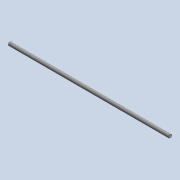
# Autodesk Inventor part: SFR6-284
Saved by Autodesk Inventor 2022 (Build 260153000, 153)
## iProperties
Part Number: SFR6-284
Material: 一般
Catalog Web Link: www.cadenas.de
Description: NSFMR, SFMR, PSFMR, SSFMR, SSSFMR, NSFHR, SFHR, PSFHR, PPSFHR SSFHR, SSSFHR, NSFR, SFR, PSFR, PPSFR, SSFR, SSSFR, HFR, PHFR_shaft-Rotary Shafts - Straight -
Vendor: MISUMI
Document SubType Name: Modeling
Designer: partserver
Manufacturer: MISUMI
Mass: 8.02546 g
Surface Area: 53.9813 cm^2
Volume: 8.02546 cm^3
Density: 1 g/cm^3
Appearance: PSOLRGB-192-192-192
Category: PARTsolutions
Company: MISUMI
PSOL_IDENT_0: {$CADENAS_DATA\23d-libs\misumi\metric\11_rotary_shafts\11_components\psfr\psfr.prj},557 {VTYP=3D},{N
PSOL_IDENT_1: B=SFR6-284(000_000)_s},{LINA=SFR6-284},{NN=NSFMR, SFMR, PSFMR, SSFMR, SSSFMR, NSFHR, SFHR, PSFHR, PP
PSOL_IDENT_2: SFHR SSFHR, SSSFHR, NSFR, SFR, PSFR, PPSFR, SSFR, SSSFR, HFR, PHFR_shaft},{DATE=27.07.2021 07:07:26}
PSOL_IDENT_3: ,{GEOMDATE=27.07.2021 07:07:13},{VERSION=},{LINEID=110},{WBVAR=TS,MAT,ST,ALT1,L,ALT2,KC,A,WKC,C,K,E,
PSOL_IDENT_4: KZ,Z,ALT3,FC,GALT3,WFC,J,WALT3,V,ALT4,SFC,SG,AG,ALT10,KWC,ALT11,WC,ALT6,TA,TB,ALT5,UC,ALT7,SC,ALT32,
PSOL_IDENT_5: CD,ALT34,TCJ,WTCJ,XT,HCJ,WHCJ,XH},{WBNUMERIC=L,KC,A,WKC,C,K,E,KZ,Z,FC,GALT3,WFC,J,WALT3,V,SFC,SG,AG,
PSOL_IDENT_6: KWC,WC,TA,TB,UC,SC,TCJ,WTCJ,XT,HCJ,WHCJ,XH}  {NB=SFR6-284(000_000)_s},{LINA=SFR6-284},{KT=DUMMY},{PN=
PSOL_IDENT_7: SFR6-284},{TYPE=SFR},{TS=},{TSALG= 'M','h9 (Cold-drawn)','H','h7 (Ground)','','g6 (Ground)' },{MAT=S
PSOL_IDENT_8: 45C},{MATALG= 'S45C','S45C Equivalent', 'SUS304','304 Stainless Steel','SUS303','303 Stainless Steel'
PSOL_IDENT_9: },{ST=BO},{STALG= '','-','BO','Black Oxide', 'ENP','Electroless Nickel Plating', 'HCP','Hard chrome
PSOL_IDENT_10: plating' },{D=6.0},{ALT1=},{L=284.0},{LALG=[15:500/0.1]},{LMIN=15},{LMAX=500},{NOTE=Not Applicable}
PSOL_IDENT_11: ,{ALT2=},{ALT2ALG= '', 'w/o Key Grooves','KC','with KC (Key Groove)','WKC','with WKC (Two Key Groove
PSOL_IDENT_12: s)','KCWKC','with KC + WKC (Three Key Grooves)','KZ','with KC + WKC + KZ (Four Key Grooves)' },{ALT2
PSOL_IDENT_13: PN=},{KC=0.0},{KCALG=[0]},{KCMIN=0},{KCMAX=0},{A=0.0},{AALG=[0]},{AMIN=2},{AMAX=0},{WKC=0.0},{WKCALG=
PSOL_IDENT_14: [0]},{WKCMIN=0},{WKCMAX=0},{C=0.0},{CALG=[0]},{CMIN=2},{CMAX=0},{K=0.0},{KALG=[0]},{KMIN=0},{KMAX=28
PSOL_IDENT_15: 0},{E=0.0},{EALG=[0]},{EMIN=2},{EMAX=100},{KZ=0.0},{KZALG=[0]},{KZMIN=286},{KZMAX=282},{Z=0.0},{ZALG=
PSOL_IDENT_16: [0]},{ZMIN=2},{ZMAX=100},{CIFKC=1},{CIFWKC=1},{CIFK=1},{CIFKZ=2},{PCUT3D=0.000},{QCUT3D=0},{BB=2},{B
PSOL_IDENT_17: BALT2=2},{TT=1.2},{TTALT2=1.2},{ALT3=},{ALT3ALG= '', 'w/o Set Screw Flat','FC','with FC (Adds a Set
PSOL_IDENT_18: Screw Flat)','WFC','with WFC (Adds Two Set Screw Flats)','FCWFC','with FC + WFC (Adds Three Set Scre
PSOL_IDENT_19: w Flats)' },{ALT3PN=},{FC=0},{FCALG=[0]},{FCMIN=0},{FCMAX=283},{GALT3=0},{GALT3ALG=[0]},{GALT3MIN=1}
PSOL_IDENT_20: ,{GALT3MAX=70},{GALT3MAX2=70},{GALT3MAX3=70},{WFC=0},{WFCALG=[0]},{WFCMIN=0},{WFCMIN2=2},{WFCMAX=280
PSOL_IDENT_21: },{WFCMAX2=-3},{WFCMAX3=-4},{J=0},{JALG=[0]},{JMIN=1},{JMAX=70},{JMAX2=-2},{JMAX3=-5},{WALT3=0},{WAL
PSOL_IDENT_22: T3ALG=[0]},{WALT3MIN=0},{WALT3MIN2=286},{WALT3MAX=281},{WALT3MAX2=281},{WALT3MAX3=281},{V=0},{VALG=[
PSOL_IDENT_23: 0]},{VMIN=1},{VMAX=70},{VMAX2=70},{VMAX3=50},{CIFFC=0},{ALT4=},{ALT4ALG= '', 'w/o SFC (2 Set Screw F
PSOL_IDENT_24: lats (Angle Specified))', 'SFC'  , 'with SFC (2 Set Screw Flats (Angle Specified))'},{ALT4PN=},{SFC=
PSOL_IDENT_25: 0},{SFCALG=[0]},{SFCMIN=0},{SFCMAX=283},{SG=0},{SGALG=[0]},{SGMIN=1},{SGMAX=70},{AG=0},{AGALG=[0]},{
PSOL_IDENT_26: H=0.0},{CIFSFC=0},{ALT10=},{ALT10ALG= '','Not applicable' },{ALT10PN=},{KWC=0},{KWCALG=[0]},{KWCMIN=
PSOL_IDENT_27: 1},{KWCMAX=141},{WALT10=0},{ALT11=},{ALT11ALG= '','Not applicable' },{ALT11PN=},{WC=0.0},{WCALG=[0]}
PSOL_IDENT_28: ,{ALT6=},{ALT6ALG= '','w/o Retaining Ring Groove','TA','with TA (Retaining Ring Groove)','TB','with
PSOL_IDENT_29: TB (Retaining Ring Groove)','TATB','with TA + TB (Two Retaining Ring Grooves)' },{ALT6PN=},{TA=0.0},
PSOL_IDENT_30: {TAALG=[0]},{TAMIN=2},{TAMAX=0},{TB=0.0},{TBALG=[0]},{TBMIN=2},{TBMAX=0},{DDALT6=0.0},{MM=0.00},{ALT
PSOL_IDENT_31: 5=},{ALT5ALG= '', 'w/o UC (Slit Cam Groove)', 'UC', 'with UC (Slit Cam Groove)'},{ALT5PN=},{UC=0},{U
PSOL_IDENT_32: CALG=[0]},{UCMIN=1},{UCMAX=279},{DDALT5=0},{LL1=0},{ALT7=},{ALT7ALG= '', 'w/o SC (Wrench Flats)', 'S
PSOL_IDENT_33: C', 'with SC (Wrench Flats)'},{ALT7PN=},{SC=0},{SCALG=[0]},{SCMIN=0},{SCMAX=276},{WALT7=0},{LL2=0},{
PSOL_IDENT_34: LL2ALG=8},{CIFSC=0},{ALT32=},{ALT32ALG=  '','w/o CD (Changes Part D Chamfering)','-CD', 'with CD (Ch
PSOL_IDENT_35: anges Part D Chamfering)' },{ALT32PN=},{CD=},{CDALG= '','N/A' },{CD3D=0.5},{CIF32=0},{CIF320=0},{CIF
PSOL_IDENT_36: TA=0},{CIFTB=0},{ERRORPN=},{ERRORALT23=OK},{ERRORALT24=OK},{ERRORALT25=OK},{ERRORALT26=OK},{ERRORALT
PSOL_IDENT_37: 27=OK},{ERRORALT210=OK},{ERRORALT34=OK},{ERRORALT35=OK},{ERRORALT36=OK},{ERRORALT37=OK},{ERRORALT310=
PSOL_IDENT_38: OK},{ERRORALT45=OK},{ERRORALT46=OK},{ERRORALT47=OK},{ERRORALT410=OK},{ERRORALT56=OK},{ERRORALT57=OK}
PSOL_IDENT_39: ,{ERRORALT510=OK},{ERRORALT610=OK},{ERRORALT75=OK},{ERRORALT76=OK},{ERRORALT710=OK},{ALT34=},{ALT34A
PSOL_IDENT_40: LG= '','Not applicable'},{TCJ=0},{WTCJ=0},{XT=0},{TM=0},{TCJALG=[0]},{TCJMIN=0.000},{TCJMAX=0.000},{
PSOL_IDENT_41: TCJMAX1=141.000},{HCJ=0},{WHCJ=0},{XH=0},{HP=0},{HCJALG=[0]},{HCJMIN=0.000},{HCJMAX=0.000},{HCJMAX1=
PSOL_IDENT_42: 141.000},{LCJ=0},{LMINX=0},{XCJMIN=0.000},{XALG=[0]},{XCJMAX=141.000},{WHCJMIN=0.000},{WTCJMIN=0.000
PSOL_IDENT_43: },{WTCJALG=[0]},{WHCJALG=[0]},{XHCJMIN=0.000},{XHALG=[0]}
NB: SFR6-284(000_000)_s
NN: NSFMR, SFMR, PSFMR, SSFMR, SSSFMR, NSFHR, SFHR, PSFHR, PPSFHR SSFHR, SSSFHR, NSFR, SFR, PSFR, PPSFR, SSFR, SSSFR, HFR, PHFR_shaft
NT: Rotary Shafts - Straight -
NBSYN: $PN.($ALT34.$TCJ.$WTCJ.$XT._$HCJ.$WHCJ.$XH.)_s
LINA: SFR6-284
CATALOG: Misumi
PN: SFR6-284
TS: g6 (Ground)
MAT: S45C Equivalent
ST: Black Oxide
D: 6
ALT1: w/o LKC (Changes L Tolerance)
L: 284
ALT2: w/o Key Grooves
KC: 0
A: 0
WKC: 0
C: 0
K: 0
E: 0
KZ: 0
Z: 0
ALT3: w/o Set Screw Flat
FC: 0
GALT3: 0
WFC: 0
J: 0
WALT3: 0
V: 0
ALT4: w/o SFC (2 Set Screw Flats (Angle Specified))
SFC: 0
SG: 0
AG: 0
H: 0
ALT10: Not applicable
KWC: 0
ALT11: Not applicable
WC: 0
ALT6: w/o Retaining Ring Groove
TA: 0
TB: 0
DDALT6: 0
MM: 0
ALT5: w/o UC (Slit Cam Groove)
UC: 0
DDALT5: 0
LL1: 0
ALT7: w/o SC (Wrench Flats)
SC: 0
WALT7: 0
LL2: 0
ALT32: w/o CD (Changes Part D Chamfering)
CD: N/A
ALT34: Not applicable
TCJ: 0
WTCJ: 0
XT: 0
HCJ: 0
WHCJ: 0
XH: 0
SUPPLIER: MISUMI
ARTICLENO: SFR6-284(000_000)_s
BOMINFO: SFR6-284
CREATOR: CADENAS GmbH
Title: SFR6-284
Author: Cadenas PARTsolutions
Comments: Rotary Shafts - Straight -
Autodesk Inventor part; units mm, degrees
ref_plane "YZ Plane" through (0, 0, 0) normal (1, 0, 0) x (0, 1, 0)
ref_plane "XZ Plane" through (0, 0, 0) normal (0, 1, 0) x (-1, 0, 0)
ref_plane "XY Plane" through (0, 0, 0) normal (0, 0, 1) x (1, 0, 0)
sketch "Sketch_1" plane through (0, 0, 0) normal (0, 0, 1) x (1, 0, 0)
  line L0 (284, 0) -> (0, 0)
  line L1 (0, 0) -> (0, 2.5)
  line L2 (0, 2.5) -> (0.5, 3)
  line L3 (0.5, 3) -> (283.5, 3)
  line L4 (283.5, 3) -> (284, 2.5)
  line L5 (284, 2.5) -> (284, 0)
  line L6 (284, 0) -> (0, 0)
  constraints: 14 end point
revolve "Revolution1" add sketch "Sketch_1" angle 360 about axis through (284, 0, 0) along (1, 0, 0)
ref_plane "COMBINATION_MODULE_XY" through (0, 0, 0) normal (1, 0, 0) x (0, 0, -1)
ref_plane "COMBINATION_MODULE_YZ" through (0, 0, 0) normal (0, 0, -1) x (0, 1, 0)
ref_plane "COMBINATION_MODULE_ZX" through (0, 0, 0) normal (0, 1, 0) x (1, 0, 0)
body "Solid1"
